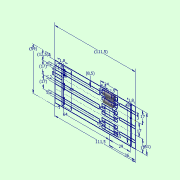
# Autodesk Inventor part: Distance_test_rig
Saved by Autodesk Inventor 2015 (Build 190159000, 159)
## iProperties
Created: 2015-05-18
Part Number: Distance_test_rig
Material: Generic
Document SubType Name: Modeling
Designer: Openlab
Density: 1 g/cm^3
Appearance: Default
Author: Openlab
Autodesk Inventor part; units mm, degrees
ref_plane "YZ Plane" through (0, 0, 0) normal (1, 0, 0) x (0, 1, 0)
ref_plane "XZ Plane" through (0, 0, 0) normal (0, 1, 0) x (-1, 0, 0)
ref_plane "XY Plane" through (0, 0, 0) normal (0, 0, 1) x (1, 0, 0)
sketch "Sketch1" plane through (0, 0, 0) normal (0, 1, 0) x (-1, 0, 0)
  line L0 (42.25, 14.75) -> (29.75, 14.75)
  line L1 (29.75, 14.75) -> (29.75, 2.25)
  line L2 (29.75, 2.25) -> (42.25, 2.25)
  line L3 (42.25, 2.25) -> (42.25, 14.75)
  line L4 (111.5, 0) -> (111.5, 17)
  line L5 (56.9183, 8.5) -> (28.9183, 8.5) construction
  line L6 (36, 15.8529) -> (36, -5.1471) construction
  line L7 (100, 15.5) -> (100, -32.5)
  line L8 (101.8, -32.5) -> (101.8, 15.5)
  line L9 (50, 11.1) -> (111.5, 11.1)
  line L10 (111.5, 5.9) -> (50, 5.9)
  line L11 (7, 15.5) -> (7, -32.5)
  line L12 (5.2, 15.5) -> (5.2, -32.5)
  line L13 (0, 17) -> (0, 0)
  line L14 (48, 7) -> (42.25, 7)
  line L15 (42.25, 10) -> (48, 10)
  line L16 (29.75, 7) -> (24, 7)
  line L17 (24, 10) -> (29.75, 10)
  line L18 (42.25, 2.25) -> (46.45, 2.25)
  line L19 (46.45, 2.25) -> (46.45, 5.45)
  line L20 (46.45, 5.45) -> (42.25, 5.45)
  line L21 (42.25, 5.45) -> (29.75, 5.45)
  line L22 (25.15, 5.45) -> (25.15, 2.25)
  line L23 (25.15, 2.25) -> (28.35, 2.25)
  line L24 (28.35, 5.45) -> (25.15, 5.45)
  line L25 (28.35, 14.75) -> (25.15, 14.75)
  line L26 (25.15, 14.75) -> (25.15, 11.55)
  line L27 (25.15, 11.55) -> (28.35, 11.55)
  line L28 (29.75, 11.55) -> (42.25, 11.55)
  line L29 (46.45, 11.55) -> (46.45, 14.75)
  line L30 (42.25, 14.75) -> (46.45, 14.75)
  line L31 (46.45, 11.55) -> (42.25, 11.55)
  line L32 (28.35, 2.25) -> (28.35, 5.45)
  line L33 (28.35, 11.55) -> (28.35, 14.75)
  line L34 (29.75, 2.25) -> (28.35, 2.25)
  line L35 (29.75, 5.45) -> (28.35, 5.45)
  line L36 (29.75, 11.55) -> (28.35, 11.55)
  line L37 (29.75, 14.75) -> (28.35, 14.75)
  line L38 (111.5, 17) -> (0, 17)
  line L39 (22, 10) -> (0, 10)
  line L40 (22, 7) -> (0, 7)
  line L41 (0, 0) -> (111.5, 0) construction
  line L42 (100, 12.5) -> (98.2, 12.5)
  line L43 (98.2, 12.5) -> (98.2, 4.5)
  line L44 (98.2, 4.5) -> (100, 4.5)
  line L45 (0, 0) -> (0, -34)
  line L46 (0, -17) -> (111.5, -17) construction
  line L47 (111.5, -34) -> (111.5, 0)
  line L48 (42.25, -2.25) -> (29.75, -2.25)
  line L49 (29.75, -2.25) -> (29.75, -14.75)
  line L50 (29.75, -14.75) -> (42.25, -14.75)
  line L51 (42.25, -14.75) -> (42.25, -2.25)
  line L52 (56.8064, -8.5) -> (28.8064, -8.5) construction
  line L53 (36, 2.2048) -> (36, -34) construction
  line L54 (48, -10) -> (42.25, -10)
  line L55 (42.25, -7) -> (48, -7)
  line L56 (42.25, -14.75) -> (46.45, -14.75)
  line L57 (46.45, -14.75) -> (46.45, -11.55)
  line L58 (46.45, -11.55) -> (42.25, -11.55)
  line L59 (42.25, -11.55) -> (29.75, -11.55)
  line L60 (25.15, -11.55) -> (25.15, -14.75)
  line L61 (25.15, -14.75) -> (28.35, -14.75)
  line L62 (28.35, -11.55) -> (25.15, -11.55)
  line L63 (28.35, -2.25) -> (25.15, -2.25)
  line L64 (25.15, -2.25) -> (25.15, -5.45)
  line L65 (25.15, -5.45) -> (28.35, -5.45)
  line L66 (29.75, -5.45) -> (42.25, -5.45)
  line L67 (46.45, -5.45) -> (46.45, -2.25)
  line L68 (42.25, -2.25) -> (46.45, -2.25)
  line L69 (46.45, -5.45) -> (42.25, -5.45)
  line L70 (28.35, -14.75) -> (28.35, -11.55)
  line L71 (28.35, -5.45) -> (28.35, -2.25)
  line L72 (29.75, -14.75) -> (28.35, -14.75)
  line L73 (29.75, -11.55) -> (28.35, -11.55)
  line L74 (29.75, -5.45) -> (28.35, -5.45)
  line L75 (29.75, -2.25) -> (28.35, -2.25)
  line L76 (50, -5.9) -> (111.5, -5.9)
  line L77 (111.5, -11.1) -> (50, -11.1)
  line L78 (100, -4.5) -> (98.2, -4.5)
  line L79 (98.2, -4.5) -> (98.2, -12.5)
  line L80 (98.2, -12.5) -> (100, -12.5)
  line L81 (0, -34) -> (111.5, -34)
  line L82 (42.25, -28.55) -> (29.75, -28.55)
  line L83 (29.75, -22.45) -> (42.25, -22.45)
  line L84 (29.75, -19.25) -> (29.75, -31.75)
  line L85 (42.25, -19.25) -> (29.75, -19.25)
  line L86 (42.25, -31.75) -> (42.25, -19.25)
  line L87 (29.75, -31.75) -> (42.25, -31.75)
  line L88 (42.25, -31.75) -> (46.45, -31.75)
  line L89 (46.45, -31.75) -> (46.45, -28.55)
  line L90 (46.45, -28.55) -> (42.25, -28.55)
  line L91 (46.45, -22.45) -> (42.25, -22.45)
  line L92 (42.25, -19.25) -> (46.45, -19.25)
  line L93 (46.45, -22.45) -> (46.45, -19.25)
  line L94 (29.75, -28.55) -> (28.35, -28.55)
  line L95 (29.75, -31.75) -> (28.35, -31.75)
  line L96 (28.35, -31.75) -> (28.35, -28.55)
  line L97 (29.75, -22.45) -> (28.35, -22.45)
  line L98 (29.75, -19.25) -> (28.35, -19.25)
  line L99 (28.35, -22.45) -> (28.35, -19.25)
  line L100 (25.15, -31.75) -> (28.35, -31.75)
  line L101 (25.15, -28.55) -> (25.15, -31.75)
  line L102 (28.35, -28.55) -> (25.15, -28.55)
  line L103 (25.15, -22.45) -> (28.35, -22.45)
  line L104 (28.35, -19.25) -> (25.15, -19.25)
  line L105 (25.15, -19.25) -> (25.15, -22.45)
  line L106 (56.4151, -25.5) -> (28.8749, -25.5) construction
  line L107 (50, -22.9) -> (111.5, -22.9)
  line L108 (111.5, -28.1) -> (50, -28.1)
  line L109 (100, -21.5) -> (98.2, -21.5)
  line L110 (98.2, -21.5) -> (98.2, -29.5)
  line L111 (98.2, -29.5) -> (100, -29.5)
  line L112 (42.25, -24) -> (48, -24)
  line L113 (48, -27) -> (42.25, -27)
  line L114 (101.8, 15.5) -> (100, 15.5)
  line L115 (101.8, -32.5) -> (100, -32.5)
  line L116 (7, -32.5) -> (5.2, -32.5)
  line L117 (7, 15.5) -> (5.2, 15.5)
  line L118 (111.5, -2) -> (101.8, -2)
  line L119 (101.8, 2) -> (111.5, 2)
  line L120 (48, -27) -> (48, -24)
  line L121 (50, -22.9) -> (50, -28.1)
  line L122 (50, -11.1) -> (50, -5.9)
  line L123 (48, -7) -> (48, -10)
  line L124 (50, 5.9) -> (50, 11.1)
  line L125 (48, 10) -> (48, 7)
  line L126 (24, -24) -> (24, -27)
  line L127 (22, -27) -> (22, -24)
  line L128 (0, -24) -> (22, -24)
  line L129 (24, -24) -> (29.75, -24)
  line L130 (29.75, -27) -> (24, -27)
  line L131 (22, -27) -> (0, -27)
  line L132 (24, 10) -> (24, 7)
  line L133 (24, -7) -> (24, -10)
  line L134 (22, -10) -> (22, -7)
  line L135 (22, 7) -> (22, 10)
  line L136 (0, -7) -> (22, -7)
  line L137 (24, -7) -> (29.75, -7)
  line L138 (29.75, -10) -> (24, -10)
  line L139 (22, -10) -> (0, -10)
  line L140 (134.256, 21) -> (125.256, 21) construction
  line L141 (134, -38) -> (123, -38) construction
  point P0 (101.8, 5.9)
  point P1 (100, 11.1)
  point P2 (100, 5.9)
  point P3 (7, 0)
  point P4 (5.2, 0)
  point P5 (7, 7)
  point P6 (5.2, 7)
  point P7 (5.2, 10)
  point P8 (7, 10)
  point P9 (36, 8.5)
  point P10 (98.2, 11.1)
  point P11 (98.2, 5.9)
  point P12 (36, -8.5)
  point P13 (101.8, 11.1)
  dimension "d0" = 12.5
  dimension "d1" = 12.5
  dimension "d12" = 5.2
  dimension "d78" = 3.2
  dimension "d79" = 1.4
  dimension "d80" = 3.2
  dimension "d92" = 17
  dimension "d93" = 3
  dimension "d95" = 1.8
  dimension "d96" = 4.2
  dimension "d112" = 5.2
  dimension "d117" = 17
  dimension "d118" = 17
  dimension "d121" = 1.8
  dimension "d122" = 5.2
  dimension "d125" = 8
  dimension "d127" = 1.8
  dimension "d130" = 17
  dimension "d131" = 8.5
  dimension "d132" = 51
  dimension "d133" = 111.5
  dimension "d134" = 48
  dimension "d135" = 48
  dimension "d136" = 4
  dimension "d137" = 2
  dimension "d138" = 2
  dimension "d140" = 24
  dimension "d142" = 29
  dimension "d143" = 36
  dimension "d144" = 64
  dimension "d145" = 111.5
  dimension "d146" = 4
  dimension "d147" = 12.5
  dimension "d148" = 7
  dimension "d149" = 17
  dimension "d150" = 4
  dimension "d151" = 59
  constraints: 282 end point, 103 point on line, 52 perpendicular, 36 collinear, 30 parallel, 28 horizontal, 2 coincident, 2 midpoint, 2 vertical, 39 other
  measures "d0" distance of L2.end L1.end
  measures "d1" distance of L0.end L1.end
  measures "d12" distance between parallel lines of L10 L9
  measures "d78" distance of L29.start L29.end
  measures "d79" distance between parallel lines of L32 L1
  measures "d80" distance of L22.end L23.end
  measures "d92" distance of L13.start L13.end
  measures "d93" distance between parallel lines of L40 L39
  measures "d95" distance of L43.end L44.end
  measures "d96" distance between parallel lines of L3 L29
  measures "d112" distance between parallel lines of L77 L76
  measures "d117" distance between parallel lines of L46 L41
  measures "d118" distance between parallel lines of L81 L46
  measures "d122" distance between parallel lines of L108 L107
  measures "d125" distance of L42.end L43.end
  measures "d127" distance between parallel lines of L11 L12
  measures "d130" distance between parallel lines of L52 L5
  measures "d131" distance between parallel lines of L38 L5
  measures "d132" distance between parallel lines of L81 L38
  measures "d133" distance between parallel lines of L13 L4
  measures "d134" distance between parallel lines of L115 L114
  measures "d135" distance between parallel lines of L117 L116
  measures "d136" distance between parallel lines of L119 L118
  measures "d137" distance between parallel lines of L127 L126
  measures "d138" distance between parallel lines of L121 L120
  measures "d140" distance between parallel lines of L132 L125
  measures "d142" distance between parallel lines of L11 L53
  measures "d143" distance between parallel lines of L45 L53
  measures "d145" distance between parallel lines of L45 L47
  measures "d146" distance between parallel lines of L38 L140
  measures "d147" distance between parallel lines of L140 L5
  measures "d148" distance between parallel lines of L5 L114
  measures "d149" distance between parallel lines of L106 L52
  measures "d150" distance between parallel lines of L141 L81
  measures "d151" distance between parallel lines of L140 L141
extrude "Extrusion10" [suppressed]
extrude "Extrusion11" add sketch "Sketch1" against normal blind 3 contours L3 L28 L1 L0 | L1 L36 L33 L37 | L3 L2 L1 L21 | L1 L34 L32 L35
extrude "Extrusion12" [suppressed]
extrude "Extrusion13" [suppressed]
extrude "Extrusion14" add sketch "Sketch1" along normal blind 2.5 contours L3 L28 L1 L0 | L3 L21 L1 L28 | L3 L2 L1 L21
body "Solid3"
